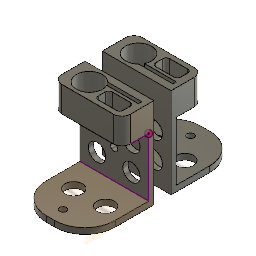
Led arch holder (Autodesk Fusion 360 design; units mm, degrees)
Autodesk Fusion 360 part; units mm, degrees
note: some values were not read from the file. Set by a fixed rule: which sketch regions a step uses.
sketch "Sketch1" plane through (0, 0, 0) normal (0, 1, 0) x (1, 0, 0) in component "Plastic"
  line L0 (20, 0) -> (20, -2)
  line L1 (20, -2) -> (0.3284, -2)
  line L2 (-1.2385, -2.7571) -> (-3.3879, -5.467)
  line L3 (-5.1399, -5.262) -> (-1.5667, -0.7571)
  line L4 (20, 0) -> (0.0002, 0)
  arc A0 (0.0002, 0) -> (-1.5667, -0.7571) centre (0.0002, -2) ccw
  arc A1 (0.3284, -2) -> (-1.2385, -2.7571) centre (0.3284, -4) ccw
  circle A2 centre (-5.1399, -5.262) radius 7.5
  dimension "d1" = 20
  dimension "d2" = 2
  dimension "d5" = 1.5
  dimension "d6" = 2
  dimension "d7" = 2
  dimension "d8" = 15
  measures "d2" distance of origin
  measures "d5" distance of L2 L3
  measures "d6" radius of A0
  measures "d7" radius of A1
  measures "d8" diameter of A2
extrude "Extrude1" add sketch "Sketch1" along normal blind 16 makes body 1 in component "Plastic"
sketch "Sketch1 (2)" plane through (0, 0, 0) normal (0, 1, 0) x (1, 0, 0) in component "Holder Left"
  line L0 (-17, 4) -> (23, 4)
  line L1 (23, 4) -> (23, -9.5)
  line L2 (18, -14.5) -> (-12, -14.5)
  line L3 (-17, -9.5) -> (-17, 4)
  arc A0 (18, -14.5) -> (23, -9.5) centre (18, -9.5) ccw
  arc A1 (-17, -9.5) -> (-12, -14.5) centre (-12, -9.5) ccw
  line L4 (6.4912, -3.6601) -> (16.9516, -3.6601)
  line L5 (18.9516, -5.6601) -> (18.9516, -9.7396)
  line L6 (16.9516, -11.7396) -> (6.4912, -11.7396)
  line L7 (4.4912, -9.7396) -> (4.4912, -5.6601)
  arc A2 (16.9516, -11.7396) -> (18.9516, -9.7396) centre (16.9516, -9.7396) ccw
  arc A3 (18.9516, -5.6601) -> (16.9516, -3.6601) centre (16.9516, -5.6601) ccw
  arc A4 (6.4912, -3.6601) -> (4.4912, -5.6601) centre (6.4912, -5.6601) ccw
  arc A5 (4.4912, -9.7396) -> (6.4912, -11.7396) centre (6.4912, -9.7396) ccw
  dimension "d15" = 5
  dimension "d16" = 5
  dimension "d18" = 2
  dimension "d19" = 2
  dimension "d20" = 2
  dimension "d21" = 2
  dimension "d49" = 40
  dimension "d50" = 23
  dimension "d51" = 18.5
  dimension "d52" = 14.5
  measures "d15" radius of A0
  measures "d16" radius of A1
  measures "d18" radius of A2
  measures "d19" radius of A3
  measures "d20" radius of A4
  measures "d21" radius of A5
  measures "d50" distance of origin L1
  measures "d51" distance of L0 L2
  measures "d52" distance of origin L2
extrude "Extrude1'" add sketch "Sketch1 (2)" along normal blind 15 separate body makes body 2 in component "Holder Left"
combine "Combine1" operation cut target body 2 tool bodies 1 keep tools in component "Holder Left"
sketch "Sketch3" plane through (0, 0, 0) normal (0, -1, 0) x (1, 0, 0) in component "Holder Left"
  line L0 (20, 2) -> (20, 0)
  line L1 (20, 0) -> (0.2043, 0)
  arc A0 (1.6135, 2) -> (0.2043, 0) centre (-5.1399, 5.262) ccw
  line L2 (1.6135, 2) -> (20, 2)
  arc A1 (4.4912, 5.6601) -> (6.4912, 3.6601) centre (6.4912, 5.6601) ccw
  line L3 (4.4912, 5.6601) -> (4.4912, 9.7396)
  arc A2 (6.4912, 11.7396) -> (4.4912, 9.7396) centre (6.4912, 9.7396) ccw
  line L4 (6.4912, 11.7396) -> (16.9516, 11.7396)
  arc A3 (18.9516, 9.7396) -> (16.9516, 11.7396) centre (16.9516, 9.7396) ccw
  line L5 (18.9516, 9.7396) -> (18.9516, 5.6601)
  arc A4 (16.9516, 3.6601) -> (18.9516, 5.6601) centre (16.9516, 5.6601) ccw
  line L6 (16.9516, 3.6601) -> (6.4912, 3.6601)
  line L7 (-17, 9.5) -> (-17, -4)
  line L8 (-17, -4) -> (23, -4)
  line L9 (23, -4) -> (23, 9.5)
  arc A5 (23, 9.5) -> (18, 14.5) centre (18, 9.5) ccw
  line L10 (18, 14.5) -> (-12, 14.5)
  arc A6 (-12, 14.5) -> (-17, 9.5) centre (-12, 9.5) ccw
  line L11 (-17, -4) -> (23, -4)
  line L12 (23, -4) -> (23, -1)
  line L13 (23, -1) -> (-17, -1)
  line L14 (-17, -1) -> (-17, -4)
  dimension "d27" = 3
extrude "Extrude2" add sketch "Sketch3" along normal blind 34 contours A0 L13 | A0 L7 L8 L9 L11 L12 L13 L14 bodies 2 in component "Holder Left"
sketch "Sketch4" plane through (0, 0, -4) normal (0, 0, -1) x (-1, 0, 0) in component "Holder Left"
  line L0 (17, -34) -> (17, 15)
  line L1 (17, 15) -> (-23, 15)
  line L2 (-23, 15) -> (-23, -34)
  line L3 (-23, -34) -> (17, -34)
  line L4 (-23, -34) -> (17, -34)
  line L5 (17, -34) -> (17, -37.5)
  line L6 (17, -37.5) -> (-23, -37.5)
  line L7 (-23, -37.5) -> (-23, -34)
  line L8 (17, 15) -> (17, -34)
  line L9 (17, -34) -> (-23, -34)
  line L10 (-23, -34) -> (-23, 15)
  dimension "d30" = 3.5
extrude "Extrude3" add sketch "Sketch4" against normal blind 40 contours L3 L4 L5 L6 L7 L9 bodies 2 in component "Holder Left"
sketch "Sketch5" plane through (23, 0, 0) normal (1, 0, 0) x (0, 0, -1) in component "Holder Left"
  line L0 (4, -37.5) -> (4, 15)
  line L1 (4, 15) -> (-9.5, 15)
  line L2 (-9.5, 15) -> (-9.5, 0)
  line L3 (1, -34) -> (-36, -34)
  line L4 (-36, -34) -> (-36, -37.5)
  line L5 (-36, -37.5) -> (4, -37.5)
  line L6 (-9.5, 0) -> (1, 0)
  line L7 (1, 0) -> (1, -34)
fillet "Fillet1" radius 17.5 2 edges at (-17, -35.75, 36) (23, -35.75, 36) on bodies 2 in component "Holder Left"
hole "Hole1" at (2.325, -37.5, 28.0383) direction (0, 1, 0) diameter 4 depth 15 tip angle 118 bodies 2 in component "Holder Left"
sketch "Sketch6" plane through (0, 0, -1) normal (0, 0, 1) x (1, 0, 0) in component "Holder Left"
  line L0 (23, 0) -> (-1.0123, 0)
  line L1 (23, -34) -> (23, 0)
  circle A0 centre (-7, -9.443) radius 5
  circle A1 centre (13, -9.443) radius 5
  circle A2 centre (13, -24.443) radius 5
  circle A3 centre (-7, -24.443) radius 5
  line L2 (18, 0) -> (-12, 0)
  circle A4 centre (3, -17) radius 2
  line L3 (-17, 0) -> (-17, -34)
  line L4 (-1.0123, 0) -> (-9.2675, 0)
  line L5 (-17, -34) -> (23, -34)
  line L6 (-9.2675, 0) -> (-17, 0)
  line L7 (23, -17) -> (-17, -17) construction
  line L8 (3, -34) -> (3, 0) construction
  line L9 (13, 0) -> (13, -34)
  line L10 (-7, 0) -> (-7, -34)
  dimension "d37" = 10
  dimension "d38" = 10
  dimension "d39" = 10
  dimension "d40" = 10
  dimension "d47" = 4
  dimension "d53" = 10
  dimension "d54" = 10
  measures "d37" diameter of A0
  measures "d38" diameter of A1
  measures "d39" diameter of A2
  measures "d40" diameter of A3
  measures "d47" diameter of A4
  measures "d53" distance of L8 L10
  measures "d54" distance of L8 L9
extrude "Extrude4" cut sketch "Sketch6" against normal blind 4 contours A1 L9 | A1 L9 | A2 L9 | A2 L9 | A3 L10 | A3 L10 | A0 L10 | A0 L10 | A4 bodies 2 in component "Holder Left"
sketch "Sketch7" plane through (0, -34, 0) normal (0, 1, 0) x (-1, 0, 0) in component "Holder Left"
  circle A0 centre (-2.325, 28.0383) radius 2
  arc A1 (-5.5, 36) -> (-23, 18.5) centre (-5.5, 18.5) ccw
  line L0 (-23, 18.5) -> (-23, -1)
  line L1 (17, -1) -> (17, 18.5)
  arc A2 (17, 18.5) -> (-0.5, 36) centre (-0.5, 18.5) ccw
  line L2 (-0.5, 36) -> (-5.5, 36)
  line L3 (-23, -1) -> (17, -1)
sketch "Sketch8" plane through (0, -37.5, 0) normal (0, -1, 0) x (1, 0, 0) in component "Holder Left"
  circle A0 centre (2.325, 28.0383) radius 2
  arc A1 (23, 18.5) -> (5.5, 36) centre (5.5, 18.5) ccw
  line L0 (5.5, 36) -> (0.5, 36)
  arc A2 (0.5, 36) -> (-17, 18.5) centre (0.5, 18.5) ccw
  line L1 (-17, 18.5) -> (-17, -4)
  line L2 (-17, -4) -> (23, -4)
  line L3 (23, -4) -> (23, 18.5)
  circle A3 centre (-4.9669, 14.5) radius 5
  line L4 (-12, 14.5) -> (18, 14.5)
  line L5 (18, 14.5) -> (-12, 14.5)
  circle A4 centre (13.0331, 14.0103) radius 5
  dimension "d43" = 10
  dimension "d44" = 10
  measures "d43" diameter of A3
  measures "d44" diameter of A4
extrude "Extrude5" cut sketch "Sketch8" against normal blind 6 contours A3 L4 L5 | A3 L4 L5 | A4 bodies 2 in component "Holder Left"
mirror "Mirror1" about plane through (0, 0, -4) normal (0, 0, -1) of bodies 2 makes body 3 in component "Holder Left"
move_body "Move1" bodies 3 to x (1, 0, 0) y (0, 1, 0) z (0, 0, 1) at (0, 0, -10) in component "Holder Left"
copy_body "CutPasteBodies1" bodies 3 removing the originals makes body 4 in component "Holder Right"
component "Plastic" placed x (1, 0, 0) y (0, 1, 0) z (0, 0, 1) at (0, 0, 0)
component "Holder Left" placed x (1, 0, 0) y (0, 1, 0) z (0, 0, 1) at (0, 0, 0)
component "Holder Right" placed x (1, 0, 0) y (0, 1, 0) z (0, 0, 1) at (0, 0, 0)
